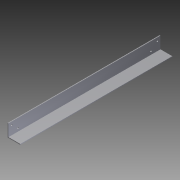
# Autodesk Inventor part: 8 ball front L
Saved by Autodesk Inventor 2012 (Build 160160000, 160)
## iProperties
Created: 2013-10-10
Part Number: 8 ball front L
Material: Default
Document SubType Name: Modeling
Designer: Bryce
Density: 1 g/cm^3
Author: Bryce
Autodesk Inventor part; units mm, degrees
ref_plane "YZ Plane" through (0, 0, 0) normal (1, 0, 0) x (0, 1, 0)
ref_plane "XZ Plane" through (0, 0, 0) normal (0, 1, 0) x (-1, 0, 0)
ref_plane "XY Plane" through (0, 0, 0) normal (0, 0, 1) x (1, 0, 0)
sketch "Sketch1" plane through (0, 0, 0) normal (0, 0, 1) x (1, 0, 0)
  line L0 (0, 0) -> (25.4, 0)
  line L1 (25.4, 0) -> (25.4, 1.5875)
  line L2 (1.5875, 25.4) -> (0, 25.4)
  line L3 (0, 25.4) -> (0, 0)
  line L4 (1.5875, 25.4) -> (1.5875, 1.5875)
  line L5 (1.5875, 1.5875) -> (25.4, 1.5875)
  dimension "d0" = 25.4
  dimension "d1" = 25.4
  dimension "d2" = 1.5875
  dimension "d3" = 1.5875
  constraints: 12 end point, 2 parallel, 1 horizontal, 1 perpendicular
  measures "d0" distance of L0.start L0.end
  measures "d1" distance of L2.end L0.start
  measures "d2" distance between parallel lines of L3 L4
  measures "d3" distance between parallel lines of L0 L5
extrude "Extrusion1" add sketch "Sketch1" along normal blind 304.8
sketch "Sketch3" plane through (0, 0, 0) normal (-1, 0, 0) x (0, 0, 1)
  line L0 (304.8, 0) -> (304.8, 25.4) projected
  line L1 (0, 25.4) -> (304.8, 25.4) projected
  line L2 (0, 0) -> (304.8, 0) projected
  circle A0 centre (298.45, 19.05) radius 1.5875
  circle A1 centre (285.75, 7.9375) radius 1.5875
  line L3 (152.4, 25.4) -> (152.4, 0) construction
  circle A2 centre (6.35, 19.05) radius 1.5875
  circle A3 centre (19.05, 7.9375) radius 1.5875
  dimension "d19" = 6.35
  dimension "d20" = 6.35
  dimension "d21" = 7.9375
  dimension "d22" = 19.05
  dimension "d23" = 3.175
  constraints: 4 centre point, 2 end point, 2 midpoint, 2 symmetric about line, 1 equal radius, 2 other
  measures "d19" distance from line of L0 A0.centre
  measures "d20" distance from line of L1 A0.centre
  measures "d21" distance from line of L2 A1.centre
  measures "d22" distance from line of L0 A1.centre
  measures "d23" diameter of A0
extrude "Extrusion4" cut sketch "Sketch3" against normal blind 25.4
equation "\"d2\" = d3"
equation "\"d20\" = d19"
body "Solid1"
